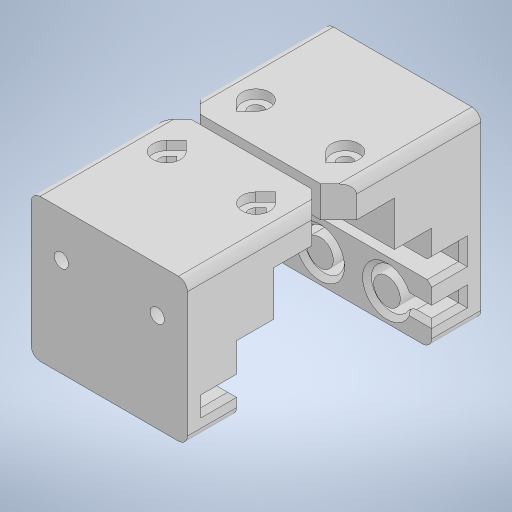
# Autodesk Inventor part: carriage
Saved by Autodesk Inventor 2023.1 (Build 271208000, 208)
## iProperties
Created: 2022-11-02
Part Number: carriage
Material: Generic
Document SubType Name: Modeling
Designer: nicol
Density: 1 g/cm^3
Appearance: Default
Author: nicol
Autodesk Inventor part; units mm, degrees
ref_plane "YZ Plane" through (0, 0, 0) normal (1, 0, 0) x (0, 1, 0)
ref_plane "XZ Plane" through (0, 0, 0) normal (0, 1, 0) x (-1, 0, 0)
sketch "Sketch1" plane through (0, 0, 0) normal (0, 1, 0) x (-1, 0, 0)
  line L0 (0, 0) -> (35, 0)
  line L1 (35, 0) -> (35, -65.7)
  line L2 (35, -65.7) -> (0, -65.7)
  line L3 (0, -65.7) -> (0, 0)
  line L4 (27.5, -22.85) -> (7.5, -22.85) construction
  line L5 (7.5, -22.85) -> (7.5, -42.85) construction
  line L6 (7.5, -42.85) -> (27.5, -42.85) construction
  line L7 (27.5, -42.85) -> (27.5, -22.85) construction
  line L8 (0, -19.35) -> (35, -19.35)
  line L9 (35, -19.35) -> (35, -46.35)
  line L10 (35, -46.35) -> (0, -46.35)
  line L11 (0, -46.35) -> (0, -19.35)
  point P0 (35, -32.85)
  point P1 (0, -46.35)
  dimension "d0" = 20
  dimension "d1" = 20
  dimension "d2" = 22.85
  dimension "d3" = 22.85
  dimension "d4" = 35
  dimension "d5" = 7.5
  dimension "d6" = 7.5
  dimension "d291" = 65.7
  dimension "d302" = 27
  constraints: 24 end point, 6 parallel, 3 horizontal, 3 perpendicular, 2 midpoint, 2 point on line
  measures "d0" distance of L6.end L5.end
  measures "d1" distance of L5.end L4.end
  measures "d2" distance between parallel lines of L0 L4
  measures "d3" distance between parallel lines of L2 L6
  measures "d4" distance of L0.start L0.end
  measures "d5" distance between parallel lines of L1 L7
  measures "d6" distance between parallel lines of L3 L5
  measures "d291" distance of L2.end L0.start
  measures "d302" distance between parallel lines of L8 L10
extrude "Extrusion1" add sketch "Sketch1" against normal blind 7
hole "Hole1" at (-27.5, 0, -22.85) at (-7.5, 0, -22.85) at (-27.5, 0, -42.85) at (-7.5, 0, -42.85) direction (0, -1, 0) diameter 3.2 end through all
sketch "Sketch2" plane through (0, -7, 0) normal (0, -1, 0) x (1, 0, 0)
  circle A0 centre (-27.5, -42.85) radius 1.6 projected
  circle A1 centre (-27.5, -22.85) radius 1.6 projected
  circle A2 centre (-7.5, -22.85) radius 1.6 projected
  circle A3 centre (-7.5, -42.85) radius 1.6 projected
  line L0 (-35, -65.7) -> (0, -65.7) projected
  line L1 (0, -65.7) -> (0, 0) projected
  line L2 (0, 0) -> (-35, 0) projected
  line L3 (-35, 0) -> (-35, -65.7) projected
  line L4 (0, -54.7) -> (-35, -54.7)
  line L5 (-35, -65.7) -> (-35, 0) projected
  line L6 (-35, -11) -> (0, -11)
  line L7 (0, 0) -> (0, -65.7) projected
  point P0 (0, -11)
  dimension "d16" = 11
  dimension "d17" = 11
  constraints: 4 end point, 4 point on line, 1 horizontal, 1 parallel
  measures "d16" distance between parallel lines of L2 L6
  measures "d17" distance between parallel lines of L0 L4
extrude "Extrusion2" add sketch "Sketch2" along normal blind 33.5 contours L3 L4 L1 L0
extrude "Extrusion24" add sketch "Sketch2" along normal blind 25 contours L3 L2 L1 L6
extrude "Extrusion28" add sketch "Sketch1" against normal blind 10 from surface at -7 contours L0 L1 L8 L3 | L10 L1 L2 L3
sketch "Sketch26" plane through (-35, -2, -11) normal (0, 0, 1) x (1, 0, 0)
  circle A0 centre (12, -23.75) radius 4.5
  circle A1 centre (12, -23.75) radius 3
  circle A2 centre (23, -23.75) radius 4.5
  circle A3 centre (23, -23.75) radius 3
  line L0 (0, -22.5) -> (12, -22.5)
  line L1 (12, -22.5) -> (12, -25)
  line L2 (12, -25) -> (0, -25)
  line L3 (0, -25) -> (0, -22.5)
  line L4 (35, -22.5) -> (23, -22.5)
  line L5 (23, -22.5) -> (23, -25)
  line L6 (23, -25) -> (35, -25)
  line L7 (35, -25) -> (35, -22.5)
  line L8 (0, 2) -> (0, -30) projected
  line L9 (35, 2) -> (35, -30) projected
  line L10 (25.9, 2) -> (29.1, 2) projected
  line L11 (9.1, -5) -> (5.9, -5) projected
  line L12 (9.1, -5) -> (5.9, -5) projected
  line L13 (29.1, -5) -> (25.9, -5) projected
  line L14 (29.1, -5) -> (25.9, -5) projected
  line L15 (0, -5) -> (35, -5) projected
  line L16 (35, -5) -> (0, -5) projected
  point P0 (9.1, -5)
  point P1 (5.9, -5)
  point P2 (29.1, -5)
  point P3 (25.9, -5)
  point P4 (27.3229, -22.5)
  point P5 (27.3229, -25)
  point P6 (7.6771, -22.5)
  point P7 (7.6771, -25)
  dimension "d264" = 2.5
  dimension "d266" = 6
  dimension "d267" = 9
  dimension "d268" = 12
  constraints: 16 end point, 5 collinear, 4 centre point, 4 coincident, 4 parallel, 2 equal radius, 2 horizontal, 2 midpoint, 2 perpendicular
  measures "d264" distance between parallel lines of L2 L0
  measures "d266" diameter of A1
  measures "d267" diameter of A0
  measures "d268" distance of L0.start L0.end
extrude "Extrusion25" cut sketch "Sketch26" along normal blind 7 contours A0 L2 A1 L0 | L7 L6 A2 L4 | L0 A1 L2 A0 | A0 L2 L3 L0 | L4 A3 L6 A2 | A2 L6 A3 L4
chamfer "Chamfer7" distance 1 angle 45 12 edges at (-3.8385, -24.5, -11) (-16.5, -25.75, -11) (-3.8385, -27, -11) (-18.5, -25.75, -11) (-31.1615, -24.5, -11) (-31.1615, -27, -11) (0, -24.5, -7.5) (0, -27, -7.5) (-35, -24.5, -7.5) (-35, -27, -7.5) (0, -25.75, -4) (-35, -25.75, -4)
fillet "Fillet5" radius 2 4 edges at (-7.6771, -24.5, -7.0002) (-7.6771, -27, -7.0002) (-27.3229, -24.5, -7.0002) (-27.3229, -27, -7.0002)
sketch "Sketch25" plane through (-35, -17, -54.7) normal (0, 0, 1) x (1, 0, 0)
  circle A0 centre (25, -17.25) radius 1.6
  circle A1 centre (10, -17.25) radius 1.6
  circle A2 centre (25, -17.25) radius 3
  circle A3 centre (10, -17.25) radius 3
  line L0 (25, -16) -> (35, -16)
  line L1 (35, -16) -> (35, -18.5)
  line L2 (35, -18.5) -> (25, -18.5)
  line L3 (25, -18.5) -> (25, -16) construction
  line L4 (10, -16) -> (0, -16)
  line L5 (0, -16) -> (0, -18.5)
  line L6 (0, -18.5) -> (10, -18.5)
  line L7 (10, -18.5) -> (10, -16)
  circle A4 centre (25, -17.25) radius 4.5
  line L8 (0, -6.5) -> (35, -6.5)
  line L9 (35, -6.5) -> (35, -10.5)
  line L10 (35, -10.5) -> (0, -10.5)
  line L11 (0, -10.5) -> (0, -6.5)
  circle A5 centre (10, -17.25) radius 4.5
  line L12 (35, -23.5) -> (0, -23.5) projected
  line L13 (35, 10) -> (35, -23.5) projected
  line L14 (0, 10) -> (0, -23.5) projected
  point P0 (29.3229, -16)
  point P1 (29.3229, -18.5)
  point P2 (5.6771, -18.5)
  point P3 (5.6771, -16)
  dimension "d241" = 2.5
  dimension "d242" = 3.2
  dimension "d243" = 6
  dimension "d244" = 9
  dimension "d245" = 4
  dimension "d248" = 10
  dimension "d292" = 17
  dimension "d293" = 5
  constraints: 24 end point, 7 collinear, 6 centre point, 6 coincident, 6 parallel, 3 equal radius, 3 horizontal, 3 perpendicular, 2 midpoint
  measures "d241" distance of L0.end L1.end
  measures "d242" diameter of A0
  measures "d243" diameter of A2
  measures "d244" diameter of A4
  measures "d245" distance of L8.end L9.end
  measures "d248" distance of L0.start L0.end
  measures "d292" distance between parallel lines of L12 L8
  measures "d293" distance between parallel lines of L12 L2
extrude "Extrusion23" cut sketch "Sketch25" against normal blind 7 contours L0 A4 L2 A2 | A2 L2 A4 L0 | L0 L1 L2 A4 | L10 L11 L8 L9 | L4 A5 L6 L5 | A5 L6 A3 L4 | L4 A3 L6 A5
chamfer "Chamfer8" distance 1 angle 45 18 edges at (-14.5, -34.25, -54.7) (-2.8385, -33, -54.7) (-2.8385, -35.5, -54.7) (0, -33, -58.2) (0, -35.5, -58.2) (0, -34.25, -61.7) (-35, -33, -58.2) (-35, -34.25, -61.7) (-20.5, -34.25, -54.7) (-32.1615, -33, -54.7) (-32.1615, -35.5, -54.7) (-35, -35.5, -58.2) (0, -27.5, -58.2) (0, -25.5, -61.7) (0, -23.5, -58.2) (-35, -27.5, -58.2) (-35, -23.5, -58.2) (-35, -25.5, -61.7)
sketch "Sketch14" plane through (-35, -27, 0) normal (0, 0, 1) x (1, 0, 0)
  line L0 (9.55, 15.3834) -> (6.75, 13.7668)
  line L1 (6.75, 13.7668) -> (3.95, 15.3834)
  line L2 (3.95, 15.3834) -> (3.95, 18.6166)
  line L3 (3.95, 18.6166) -> (6.75, 20.2332)
  line L4 (6.75, 20.2332) -> (9.55, 18.6166)
  line L5 (9.55, 18.6166) -> (9.55, 15.3834)
  line L6 (28.25, 13.7668) -> (25.45, 15.3834)
  line L7 (25.45, 15.3834) -> (25.45, 18.6166)
  line L8 (25.45, 18.6166) -> (28.25, 20.2332)
  line L9 (28.25, 20.2332) -> (31.05, 18.6166)
  line L10 (31.05, 18.6166) -> (31.05, 15.3834)
  line L11 (31.05, 15.3834) -> (28.25, 13.7668)
  line L12 (0, 27) -> (35, 27) projected
  line L13 (0, 27) -> (0, -5) projected
  line L14 (35, 27) -> (35, -5) projected
  point P0 (6.75, 17)
  point P1 (28.25, 17)
  point P2 (0, 2.5)
  point P3 (35, 2.5)
  dimension "d120" = 5.6
  dimension "d271" = 21.5
  dimension "d274" = 10
  dimension "d275" = 6.75
  dimension "d276" = 6.75
  constraints: 24 end point, 2 vertical, 1 horizontal alignment, 1 parallel, 26 other
  measures "d120" distance between parallel lines of L5 L2
  measures "d271" distance of point (28.25, 17) point (6.75, 17)
  measures "d274" distance from line of L12 point (6.75, 17)
  measures "d275" distance from line of point (6.75, 17) L13
  measures "d276" distance from line of L14 point (28.25, 17)
extrude "Extrusion12" cut sketch "Sketch14" along normal blind 15 from surface at -19.35
hole "Hole4" at (-6.75, -10, 0) at (-28.25, -10, 0) direction (0, 0, -1) diameter 3.2 depth 11
sketch "Sketch22" plane through (0, 0, 0) normal (0, 1, 0) x (1, 0, 0)
  line L0 (16.0256, 31.85) -> (-78.6573, 31.85)
  line L1 (-78.6573, 31.85) -> (-78.6573, 33.85)
  line L2 (-78.6573, 33.85) -> (16.0256, 33.85)
  line L3 (16.0256, 33.85) -> (16.0256, 31.85)
  circle A0 centre (-7.5, 22.85) radius 1.6 projected
  circle A1 centre (-7.5, 42.85) radius 1.6 projected
  line L4 (-7.5, 22.85) -> (-7.5, 42.85) construction
  point P0 (0, 0)
  point P1 (-31.3158, 31.85)
  point P2 (-7.5, 32.85)
  point P3 (16.0256, 32.85)
  dimension "d195" = 2
  constraints: 10 end point, 3 midpoint, 2 parallel, 1 horizontal, 1 horizontal alignment, 1 perpendicular, 1 vertical
  measures "d195" distance from line of point (-31.316, 31.85) L2
extrude "Extrusion20" cut sketch "Sketch22" against normal through all contours L0 L1 L2 L3
chamfer "Chamfer3" distance 4 angle 45 4 edges at (0, -3.5, -31.85) (0, -3.5, -33.85) (-35, -3.5, -31.85) (-35, -3.5, -33.85)
fillet "Fillet3" radius 2 8 edges at (0, 0, -51.775) (-35, 0, -51.775) (-35, 0, -13.925) (0, 0, -13.925) (0, -32, -5.5) (-35, -32, -5.5) (-35, -40.5, -60.2) (0, -40.5, -60.2)
sketch "Sketch24" plane through (0, 0, 0) normal (0, 1, 0) x (1, 0, 0)
  circle A0 centre (-27.5, 42.85) radius 1.6 projected
  circle A1 centre (-7.5, 42.85) radius 1.6 projected
  line L0 (-7.5, 45.1127) -> (-9.7627, 42.85)
  line L1 (-9.7627, 42.85) -> (-7.5, 40.5873)
  line L2 (-7.5, 40.5873) -> (-5.2373, 42.85)
  line L3 (-5.2373, 42.85) -> (-7.5, 45.1127)
  circle A2 centre (-7.5, 42.85) radius 1.6 projected
  line L4 (-7.5, 45.1127) -> (-7.5, 40.5873) construction
  line L5 (-9.7627, 42.85) -> (-5.2373, 42.85) construction
  line L6 (-7.5, 45.1127) -> (-4.3, 45.1127) construction
  line L7 (-27.5, 45.1127) -> (-29.7627, 42.85)
  line L8 (-29.7627, 42.85) -> (-27.5, 40.5873)
  line L9 (-27.5, 40.5873) -> (-25.2373, 42.85)
  line L10 (-25.2373, 42.85) -> (-27.5, 45.1127)
  circle A3 centre (-27.5, 42.85) radius 1.6 projected
  line L11 (-27.5, 45.1127) -> (-27.5, 40.5873) construction
  line L12 (-29.7627, 42.85) -> (-25.2373, 42.85) construction
  line L13 (-27.5, 20.5873) -> (-29.7627, 22.85)
  line L14 (-29.7627, 22.85) -> (-27.5, 25.1127)
  line L15 (-27.5, 25.1127) -> (-25.2373, 22.85)
  line L16 (-25.2373, 22.85) -> (-27.5, 20.5873)
  line L17 (-27.5, 20.5873) -> (-27.5, 25.1127) construction
  line L18 (-29.7627, 22.85) -> (-25.2373, 22.85) construction
  line L19 (-7.5, 20.5873) -> (-9.7627, 22.85)
  line L20 (-9.7627, 22.85) -> (-7.5, 25.1127)
  line L21 (-7.5, 25.1127) -> (-5.2373, 22.85)
  line L22 (-5.2373, 22.85) -> (-7.5, 20.5873)
  circle A4 centre (-7.5, 22.85) radius 1.6 projected
  line L23 (-7.5, 20.5873) -> (-7.5, 25.1127) construction
  line L24 (-9.7627, 22.85) -> (-5.2373, 22.85) construction
  circle A5 centre (-27.5, 22.85) radius 1.6 projected
  point P0 (0, 0)
  point P1 (-6.3686, 41.7186)
  point P2 (-8.6314, 41.7186)
  point P3 (-26.3686, 41.7186)
  point P4 (-28.6314, 41.7186)
  point P5 (-2, 0)
  point P6 (-33, 29.85)
  point P7 (-6.3686, 43.9814)
  point P8 (-8.6314, 43.9814)
  point P9 (-26.3686, 43.9814)
  point P10 (-28.6314, 43.9814)
  point P11 (-6.3686, 23.9814)
  point P12 (-8.6314, 23.9814)
  point P13 (-8.6314, 21.7186)
  point P14 (-6.3686, 21.7186)
  point P15 (-26.3686, 23.9814)
  point P16 (-28.6314, 23.9814)
  point P17 (-28.6314, 21.7186)
  point P18 (-26.3686, 21.7186)
  dimension "d237" = 135
  constraints: 50 end point, 9 parallel, 6 midpoint, 6 tangent, 4 perpendicular, 3 vertical, 2 centre point, 1 equal length, 1 horizontal
  measures "d237" angle of L0 L6
extrude "Extrusion22" cut sketch "Sketch24" against normal blind 10 contours L9 L8 A0 | L2 L1 A1 | A5 | L14 L15 A5 | A4 | L20 L21 A4
ref_plane "Work Plane5" through (-4, 0, -32.85) normal (0, 0, -1) x (-1, 0, 0)
fillet "Fillet6" radius 2 4 edges at (-29.3229, -33, -58.7) (-29.3229, -35.5, -58.7) (-5.6771, -35.5, -58.7) (-5.6771, -33, -58.7)
sketch "Sketch28" plane through (0, 0, 0) normal (0, 1, 0) x (1, 0, 0)
  line L0 (-33, 35.85) -> (-33, 65.7) projected
  line L1 (-31, 33.85) -> (-33, 35.85) projected
  line L2 (-31, 33.85) -> (-4, 33.85) projected
  line L3 (-2, 35.85) -> (-4, 33.85) projected
  line L4 (-2, 65.7) -> (-2, 35.85) projected
  line L5 (-2, 65.7) -> (-33, 65.7) projected
  line L6 (-6.3686, 41.7186) -> (-7.5, 40.5873) projected
  line L7 (-7.5, 40.5873) -> (-8.6314, 41.7186) projected
  arc A0 (-6.3686, 41.7186) -> (-8.6314, 41.7186) centre (-7.5, 42.85) ccw projected
  arc A1 (-26.3686, 41.7186) -> (-28.6314, 41.7186) centre (-27.5, 42.85) ccw projected
  line L8 (-26.3686, 41.7186) -> (-27.5, 40.5873) projected
  line L9 (-27.5, 40.5873) -> (-28.6314, 41.7186) projected
  line L10 (-7.5, 25.1127) -> (-6.3686, 23.9814) projected
  arc A2 (-8.6314, 23.9814) -> (-6.3686, 23.9814) centre (-7.5, 22.85) ccw projected
  line L11 (-8.6314, 23.9814) -> (-7.5, 25.1127) projected
  line L12 (-27.5, 25.1127) -> (-26.3686, 23.9814) projected
  arc A3 (-28.6314, 23.9814) -> (-26.3686, 23.9814) centre (-27.5, 22.85) ccw projected
  line L13 (-28.6314, 23.9814) -> (-27.5, 25.1127) projected
  line L14 (-2, 29.85) -> (-2, 0) projected
  line L15 (-4, 31.85) -> (-2, 29.85) projected
  line L16 (-4, 31.85) -> (-31, 31.85) projected
  line L17 (-33, 29.85) -> (-31, 31.85) projected
  line L18 (-33, 0) -> (-33, 29.85) projected
  line L19 (-33, 0) -> (-2, 0) projected
  line L20 (-9.692, 40.658) -> (-7.5, 38.4659)
  line L21 (-7.5, 38.4659) -> (-5.308, 40.658)
  arc A4 (-5.308, 40.658) -> (-9.692, 40.658) centre (-7.5, 42.85) ccw
  arc A5 (-25.308, 40.658) -> (-29.692, 40.658) centre (-27.5, 42.85) ccw
  line L22 (-25.308, 40.658) -> (-27.5, 38.4659)
  line L23 (-27.5, 38.4659) -> (-29.692, 40.658)
  line L24 (-25.308, 25.042) -> (-27.5, 27.2341)
  line L25 (-27.5, 27.2341) -> (-29.692, 25.042)
  arc A6 (-29.692, 25.042) -> (-25.308, 25.042) centre (-27.5, 22.85) ccw
  line L26 (-5.308, 25.042) -> (-7.5, 27.2341)
  line L27 (-7.5, 27.2341) -> (-9.692, 25.042)
  arc A7 (-9.692, 25.042) -> (-5.308, 25.042) centre (-7.5, 22.85) ccw
  point P0 (0, 0)
  dimension "d301" = 3.1
  constraints: 16 end point, 8 point on circle, 4 centre point, 3 equal radius, 8 other
  measures "d301" radius of A7
extrude "Extrusion27" cut sketch "Sketch28" against normal blind 2 contours A4 L21 L20 | L22 L23 A5 | A6 L25 L24 | A7 L27 L26
equation "\"d5\" = d6"
body "Solid1"
